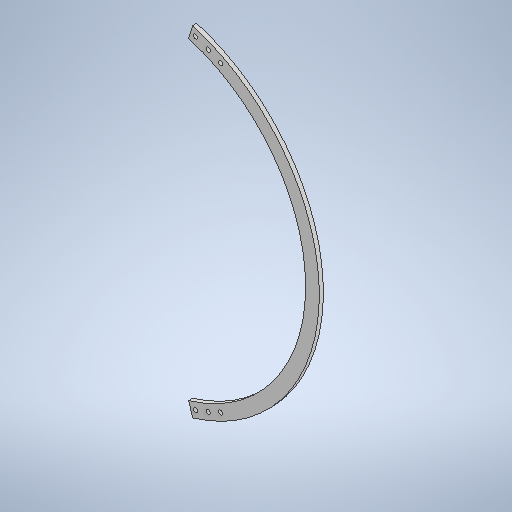
# Autodesk Inventor part: ring
Saved by Autodesk Inventor 2025.1 (Build 291241000, 241)
## iProperties
Created: 2025-05-01
Part Number: ring
Material: 一般
Document SubType Name: Modeling
Designer: yuki0520
Density: 1 g/cm^3
Appearance: 既定
Author: yuki0520
Autodesk Inventor part; units mm, degrees
ref_plane "YZ Plane" through (0, 0, 0) normal (1, 0, 0) x (0, 1, 0)
ref_plane "XZ Plane" through (0, 0, 0) normal (0, 1, 0) x (-1, 0, 0)
ref_plane "XY Plane" through (0, 0, 0) normal (0, 0, 1) x (1, 0, 0)
derived "zzz_sekkei.ipt"
sketch "スケッチ1" plane through (0, 0, 0) normal (0, 0, 1) x (1, 0, 0)
  circle A0 centre (0, 0) radius 120
  line L0 (12.25, -196) -> (-12.25, -196)
  line L1 (-12.25, -196) -> (-12.25, -120)
  line L2 (-12.25, -120) -> (12.25, -120)
  line L3 (12.25, -120) -> (12.25, -196)
  line L4 (12.25, -196) -> (-12.25, -120) construction
  line L5 (-12.25, -196) -> (12.25, -120) construction
  circle A1 centre (0, 0) radius 130
  line L6 (0, 130) -> (0, -130)
  line L7 (41.25, -164) -> (-95.75, -164)
  line L8 (-95.75, -164) -> (-95.75, -152)
  line L9 (-95.75, -152) -> (41.25, -152)
  line L10 (41.25, -152) -> (41.25, -164)
  line L11 (41.25, -164) -> (-95.75, -152) construction
  line L12 (-95.75, -164) -> (41.25, -152) construction
  line L13 (-12.25, -158) -> (12.25, -158)
  line L14 (34.25, -120) -> (34.25, -320)
  line L15 (34.25, -115.0084) -> (44.25, -115.0084)
  line L16 (44.25, -115.0084) -> (44.25, -150.0084)
  line L17 (44.25, -150.0084) -> (34.25, -150.0084)
  line L18 (34.25, -150.0084) -> (34.25, -115.0084)
  line L19 (34.25, -120) -> (44.25, -120)
  line L20 (0, 0) -> (62.2468, -114.1286)
  line L21 (0, 0) -> (37.1042, -124.5925)
  line L22 (30.3, 120) -> (-30.3, 120)
  line L23 (-30.3, 120) -> (-30.3, 138.5)
  line L24 (-30.3, 138.5) -> (30.3, 138.5)
  line L25 (30.3, 138.5) -> (30.3, 120)
  line L26 (30.3, 120) -> (-30.3, 138.5) construction
  line L27 (-30.3, 120) -> (30.3, 138.5) construction
  line L28 (34.25, 180) -> (34.25, 120)
  line L29 (34.25, 120) -> (70, 120)
  line L30 (34.25, 115.0084) -> (44.25, 115.0084)
  line L31 (44.25, 115.0084) -> (44.25, 150.0084)
  line L32 (44.25, 150.0084) -> (34.25, 150.0084)
  line L33 (34.25, 150.0084) -> (34.25, 115.0084)
  line L34 (0, 0) -> (37.1042, 124.5925)
  line L35 (0, 0) -> (62.2468, 114.1286)
  circle A2 centre (0, 0) radius 125
  point P0 (0, -158)
  point P1 (-27.25, -158)
  point P2 (0, 129.25)
  point P3 (39.25, 118.6779)
  point P4 (39.25, -118.6779)
  point P5 (34.25, -132.5084)
  point P6 (34.25, -120)
  point P7 (36.0555, -60)
  point P8 (50, 120)
  point P9 (34.25, 120)
  point P10 (35.7365, -120)
  point P11 (34.25, -125.4071)
  point P12 (44.25, -122.2372)
  point P13 (35.7365, 120)
  point P14 (44.25, 120)
  point P15 (44.25, 122.2372)
  point P16 (34.25, 125.4071)
extrude "押し出し1" add sketch "スケッチ1" along normal blind 3 contours A0 L35 A2 L20 | A0 L30 L31 A2 L35 | L20 A2 L16 L15 A0 | L34 A2 L31 L30 | A2 L31 L29 A1 L35 | L35 A1 L20 A2 | L15 L16 A2 L21 | L20 A1 L16 A2 | L34 L29 L31 A2 | A2 L16 L19 L21 | L34 A1 L31 L29 | L29 L31 A1 | L19 L16 A1 L21
sketch "スケッチ2" plane through (0, 0, 3) normal (0, 0, 1) x (1, 0, 0)
  circle A0 centre (0, 0) radius 125 projected
  line L0 (37.1042, 124.5925) -> (34.25, 115.0084) projected
  line L1 (34.25, -115.0084) -> (37.1042, -124.5925) projected
  line L2 (34.25, 150.0084) -> (34.25, 115.0084) projected
  line L3 (34.25, -150.0084) -> (34.25, -115.0084) projected
  point P0 (57.661, 110.9063)
  point P1 (48.611, 115.1606)
  point P2 (39.25, 118.6779)
  point P3 (48.611, -115.1606)
  point P4 (48.611, -115.1606)
  point P5 (39.25, -118.6779)
  point P6 (57.661, -110.9063)
  dimension "d3" = 10
  dimension "d5" = 5
  dimension "d6" = 10
  dimension "d14" = 5
  dimension "d15" = 10
  dimension "d16" = 10
  dimension "d17" = 10
  constraints: 8 other
  measures "d3" distance of point (57.661, 110.906) point (48.611, 115.161)
  measures "d5" distance from line of L2 point (39.25, 118.678)
  measures "d6" distance of point (48.611, 115.161) point (39.25, 118.678)
  measures "d14" distance from line of L3 point (39.25, -118.678)
  measures "d15" distance of point (48.611, -115.161) point (39.25, -118.678)
  measures "d16" distance of point (48.611, -115.161) point (57.661, -110.906)
  measures "d17" distance of point (57.661, -110.906) point (48.611, -115.161)
hole "穴1" at (57.661, 110.9063, 3) at (48.611, 115.1606, 3) at (48.611, -115.1606, 3) at (57.661, -110.9063, 3) at (39.25, -118.6779, 3) at (39.25, 118.6779, 3) direction (0, 0, -1) diameter 3.1 end through all
